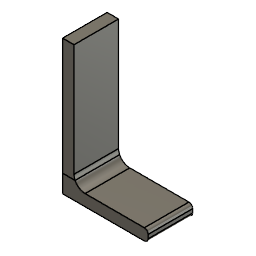
scaun (Autodesk Fusion 360 design; units mm, degrees)
part number: 2026-07-06-18-03-11-969
Autodesk Fusion 360 part; units mm, degrees
sketch "Sketch1" plane through (0, 0, 0) normal (0, 0, 1) x (1, 0, 0)
sketch "Sketch2" plane through (0, 0, 0) normal (0, 0, 1) x (1, 0, 0)
  line L0 (59.0642, 176.183) -> (193.3556, 176.183)
  line L1 (193.3556, 176.183) -> (193.3556, -35.2126)
  line L2 (193.3556, -35.2126) -> (59.0642, -35.2126)
  line L3 (59.0642, -35.2126) -> (59.0642, 176.183)
  constraint horizontal L0
  constraint vertical L1
  constraint horizontal L2
  constraint vertical L3
sketch "Sketch3" plane through (0, 0, 0) normal (0, 0, 1) x (1, 0, 0)
sketch "Sketch4" plane through (0, 0, 0) normal (0, 0, 1) x (1, 0, 0)
sketch "Sketch5" plane through (0, 0, 0) normal (0, 0, 1) x (1, 0, 0)
sketch "Sketch6" plane through (0, 0, 0) normal (0, 0, 1) x (1, 0, 0)
sketch "Sketch7" plane through (0, 0, 0) normal (0, 0, 1) x (1, 0, 0)
sketch "Sketch8" plane through (0, 0, 0) normal (0, 0, 1) x (1, 0, 0)
extrude "Extrude1" add sketch "Sketch2" along normal blind 70 makes body 1
sketch "Sketch9" plane through (0, 0, 70) normal (0, 0, 1) x (1, 0, 0)
  line L0 (59.0642, -35.2126) -> (193.3556, -35.2126)
  line L1 (193.3556, -35.2126) -> (193.3556, 176.183)
  line L2 (193.3556, 176.183) -> (59.0642, 176.183)
  line L3 (59.0642, 176.183) -> (59.0642, -35.2126)
  line L4 (59.0642, 176.183) -> (77.0642, 176.183)
  line L5 (193.3556, -35.2126) -> (193.3556, -17.2126)
  line L6 (77.0642, 176.183) -> (77.0642, -17.2126)
  line L7 (77.0642, -17.2126) -> (193.3556, -17.2126)
  dimension "d3" = 18
  dimension "d4" = 18
  constraint coincident L2.end L3.start
  constraint perpendicular L3 L4
  constraint coincident L0.end L1.start
  constraint perpendicular L0 L5
  constraint perpendicular L2 L6
  constraint perpendicular L1 L7
  measures "d3" distance of L2.end L4.end
  measures "d4" distance of L0.end L5.end
extrude "Extrude2" cut sketch "Sketch9" against normal blind 250 contours L1 L2 L6 L7 bodies 1
fillet "Fillet1" radius 17.5 1 edges at (77.0642, -17.2126, 35) on bodies 1
ref_plane "WorkPlane1" through (135.2099, -7.2126, 35) normal (0, 1, 0) x (1, 0, 0)
split "Split1" by plane through (135.2099, -7.2126, 35) normal (0, 1, 0) bodies 1 makes body 2 at (59.0642, 53.9193, 23.3333)
fillet "Fillet2" radius 6 2 edges at (193.3556, -17.2126, 35) (193.3556, -35.2126, 35) on bodies 1
